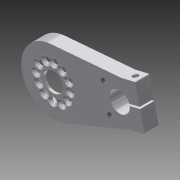
# Autodesk Inventor part: mount_alt
Saved by Autodesk Inventor 2015 SP1 (Build 190203100, 203)
## iProperties
Created: 2014-11-18
Part Number: mount_alt
Material: Aluminum 6061
Document SubType Name: Modeling
Designer: brent
Density: 2.7 g/cm^3
Appearance: Aluminum - Flat
Author: brent
Autodesk Inventor part; units mm, degrees
ref_plane "YZ Plane" through (0, 0, 0) normal (1, 0, 0) x (0, 1, 0)
ref_plane "XZ Plane" through (0, 0, 0) normal (0, 1, 0) x (-1, 0, 0)
ref_plane "XY Plane" through (0, 0, 0) normal (0, 0, 1) x (1, 0, 0)
derived "mount_sketch_alt.ipt"
sketch "Sketch2" plane through (0, 0, 0) normal (0, 0, 1) x (1, 0, 0)
  line L0 (72.4396, -72.2948) -> (-70.2441, 86.1715)
  line L1 (30.3736, -26.3701) -> (-42.626, -26.3701)
  circle A0 centre (-21.7992, 32.368) radius 3.9688
  circle A1 centre (-21.7992, 32.368) radius 9
  line L2 (-81.1368, 18.0799) -> (-21.7992, 32.368)
  circle A2 centre (-81.1368, 18.0799) radius 4
  circle A3 centre (-81.1368, 18.0799) radius 28.4798
  line L3 (-83.4978, 46.4616) -> (-7.6575, 52.7705)
  line L4 (-70.3199, -8.2657) -> (0.0796, 20.6388)
  line L5 (0.0796, 20.6388) -> (-7.6575, 52.7705)
  line L6 (-12.1479, 15.6185) -> (0.5521, 18.6766)
  line L7 (0.5521, 18.6766) -> (0.0796, 20.6388)
  line L8 (-12.8975, 33.695) -> (-3.6031, 35.933)
  line L9 (-13.2692, 35.2384) -> (-3.9747, 37.4764)
  line L10 (-88.9657, 5.285) -> (-93.9317, 25.9087)
  line L11 (-93.9317, 25.9087) -> (-73.308, 30.8748)
  line L12 (-73.308, 30.8748) -> (-68.3419, 10.251)
  line L13 (-68.3419, 10.251) -> (-88.9657, 5.285)
  line L14 (-88.9657, 5.285) -> (-73.308, 30.8748) construction
  line L15 (-93.9317, 25.9087) -> (-68.3419, 10.251) construction
  line L16 (-87.7302, 31.3952) -> (-67.3865, 25.3841)
  line L17 (-67.3865, 25.3841) -> (-73.3976, 5.0404)
  line L18 (-73.3976, 5.0404) -> (-93.7413, 11.0515)
  line L19 (-93.7413, 11.0515) -> (-87.7302, 31.3952)
  line L20 (-87.7302, 31.3952) -> (-73.3976, 5.0404) construction
  line L21 (-67.3865, 25.3841) -> (-93.7413, 11.0515) construction
  line L22 (-81.7046, 3.0401) -> (-96.3171, 18.4178)
  line L23 (-96.3171, 18.4178) -> (-80.9395, 33.0304)
  line L24 (-80.9395, 33.0304) -> (-66.3269, 17.6527)
  line L25 (-66.3269, 17.6527) -> (-81.7046, 3.0401)
  line L26 (-81.7046, 3.0401) -> (-80.9395, 33.0304) construction
  line L27 (-96.3171, 18.4178) -> (-66.3269, 17.6527) construction
  line L28 (-20.4639, 51.7052) -> (-8.1168, 54.6783)
  line L29 (-8.1168, 54.6783) -> (-7.6575, 52.7705)
  line L30 (-81.322, 18.0353) -> (-80.5639, 18.2178) construction
  line L31 (-79.3322, 9.7715) -> (-78.574, 9.954)
  line L32 (-82.5538, 26.4816) -> (-83.3119, 26.2991)
  arc A4 (-83.3119, 26.2991) -> (-79.3322, 9.7715) centre (-81.322, 18.0353) ccw
  arc A5 (-78.574, 9.954) -> (-82.5538, 26.4816) centre (-80.5639, 18.2178) ccw
  point P0 (0, 0)
  point P1 (-80.5639, 18.2178)
  point P2 (-80.943, 18.1265)
extrude "Extrusion1" add sketch "Sketch2" along normal blind 12.7 contours L6 L4 L0 | L0 L4 L7 L6 | L4 A3 L2 A1 L0 | L0 A1 L8 L5 L4 | A3 | L2 A3 L3 L0 A1 | L0 L3 L5 L9 A1 | L3 L28 L29 | L12 L24 L2 | L12 L17 L25 L13 L18 L22 L10 L19 L23 L11 L16 L24 | L2 L24 L17 L12 | L24 L12 L16 L17 L2 | L2 L17 L24 | L24 L16 L12 | L17 L24 L25 L12 | L12 L25 L17 | L16 L24 L11 L12 | L16 L11 L24 | L12 L13 L17 L25 | L17 L13 L25 | L16 L23 L24 L11 | L11 L23 L16 | L17 L18 L25 L13 | L25 L18 L13 | L23 L19 L11 | L11 L19 L16 L23 | L18 L25 L22 L13 | L13 L22 L18 | L19 L23 L10 L11 | L19 L10 L23 | L13 L10 L18 L22 | L18 L10 L22 | L19 L22 L23 L10 | L10 L22 L19 | L18 L19 L22 L10
sketch "Sketch3" plane through (-81.1368, 18.0799, 0) normal (0, 0, -1) x (-0.9722121, -0.2341019, 0)
  line L0 (-79.5587, -18.5434) -> (-79.5587, -0.7938) projected
  line L1 (-66.4957, -18.5434) -> (-79.5587, -18.5434) projected
  line L2 (-4.3488, -28.1458) -> (-66.4957, -18.5434) projected
  arc A0 (-4.3488, -28.1458) -> (-4.3488, 28.1458) centre (0, 0) ccw projected
  line L3 (-66.8587, 18.4873) -> (-4.3488, 28.1458) projected
  line L4 (-69.9986, 0.7937) -> (-79.5587, 0.7937) projected
  arc A1 (-69.9986, -0.7938) -> (-69.9986, 0.7937) centre (-61.0337, 0) ccw projected
  line L5 (-79.5587, -0.7938) -> (-69.9986, -0.7938) projected
  line L6 (0.6905, 0) -> (-0.6905, 0) construction
  line L7 (0.6905, 25.25) -> (-0.6905, 25.25)
  line L8 (-0.6905, -25.25) -> (0.6905, -25.25)
  arc A2 (0.6905, -25.25) -> (0.6905, 25.25) centre (0.6905, 0) ccw
  arc A3 (-0.6905, 25.25) -> (-0.6905, -25.25) centre (-0.6905, 0) ccw
  line L9 (-79.5587, 0.7937) -> (-79.5587, 18.4873) projected
  line L10 (-79.5587, 18.4873) -> (-66.8587, 18.4873) projected
  point P0 (-74.6497, -36.5717)
  dimension "d4" = 0.6905
  dimension "d5" = 50.5
  constraints: 8 end point, 4 point on circle, 4 tangent, 2 centre point, 1 horizontal, 1 midpoint, 1 parallel
  measures "d4" distance of A0.centre L6.end
  measures "d5" diameter of A3
extrude "Extrusion2" cut sketch "Sketch3" against normal blind 10.3188 contours A2 L8 A3 L7
hole "Hole1" at (-96.3171, 18.4178, 0) at (-93.7413, 11.0515, 0) at (-88.9657, 5.285, 0) at (-81.7046, 3.0401, 0) at (-73.3976, 5.0404, 0) at (-68.3419, 10.251, 0) at (-66.3269, 17.6527, 0) at (-67.3865, 25.3841, 0) at (-73.308, 30.8748, 0) at (-80.9395, 33.0304, 0) at (-87.7302, 31.3952, 0) at (-93.9317, 25.9087, 0) direction (0, 0, 1) diameter 4.3 end through all
sketch "Sketch4" plane through (0.5521, 18.6766, 0) normal (0.2341019, -0.9722121, 0) x (0.9722121, 0.2341019, 0)
  line L0 (-13.063, 0) -> (0, 0) projected
  line L1 (0, 0) -> (0, 12.7) projected
  line L2 (-13.063, 12.7) -> (0, 12.7) projected
  line L3 (-13.063, 0) -> (-13.063, 12.7) projected
  line L4 (-9.5601, 0) -> (-9.5601, 12.7) projected
  circle A0 centre (-6.0325, 6.35) radius 2.5527
  point P0 (-4.909, 0)
  dimension "d15" = 5.1054
  dimension "d17" = 6.0325
  dimension "d18" = 12.7
  dimension "d19" = 6.35
  constraints: 1 centre point
  measures "d15" diameter of A0
  measures "d17" distance from line of L1 A0.centre
  measures "d18" distance between parallel lines of L2 L0
  measures "d19" distance from line of L2 A0.centre
extrude "Extrusion3" cut sketch "Sketch4" against normal through all contours A0
ref_plane "Work Plane1" through (100.1901, 61.7421, 0) normal (0.2341019, -0.9722121, 0) x (0, 0, -1)
chamfer "Chamfer2" distance 2 angle 45 12 edges at (-87.7302, 29.2452, 12.7) (-80.9395, 30.8804, 12.7) (-73.308, 28.7248, 12.7) (-67.3865, 23.2341, 12.7) (-66.3269, 15.5027, 12.7) (-68.3419, 8.101, 12.7) (-73.3976, 2.8904, 12.7) (-81.7046, 0.8901, 12.7) (-88.9657, 3.135, 12.7) (-93.7413, 8.9015, 12.7) (-96.3171, 16.2678, 12.7) (-93.9317, 23.7587, 12.7)
sketch "Sketch8" plane through (-81.1368, 18.0799, 0) normal (0, 0, -1) x (-0.9722121, -0.2341019, 0)
  line L0 (-79.5587, -18.5434) -> (-79.5587, -0.7938) projected
  line L1 (-69.9986, 0.7937) -> (-79.5587, 0.7937) projected
  arc A0 (-69.9986, -0.7938) -> (-69.9986, 0.7937) centre (-61.0337, 0) ccw projected
  line L2 (-79.5587, -0.7938) -> (-69.9986, -0.7938) projected
  line L3 (-66.4957, -18.5434) -> (-79.5587, -18.5434) projected
  line L4 (-4.3488, -28.1458) -> (-66.4957, -18.5434) projected
  arc A1 (-4.3488, -28.1458) -> (-4.3488, 28.1458) centre (0, 0) ccw projected
  line L5 (-66.8587, 18.4873) -> (-4.3488, 28.1458) projected
  line L6 (-79.5587, 18.4873) -> (-66.8587, 18.4873) projected
  line L7 (-0.6905, 28.425) -> (0.6905, 28.425)
  arc A2 (0.6905, -28.425) -> (0.6905, 28.425) centre (0.6905, 0) ccw
  line L8 (0.6905, -28.425) -> (-0.6905, -28.425)
  arc A3 (-47.6803, -13.7402) -> (-47.6803, 13.7402) centre (-61.0337, 0) ccw
  line L9 (-47.6803, -13.7402) -> (-7.1186, -24.4181)
  line L10 (-47.6803, 13.7402) -> (-7.1186, 24.4181)
  arc A4 (-0.6905, 25.25) -> (-0.6905, -25.25) centre (-0.6905, 0) ccw projected
  line L11 (-79.5587, 0.7937) -> (-79.5587, 18.4873) projected
  point P0 (-74.6497, -36.5717)
  dimension "d55" = 10.16
  dimension "d91" = 7.62
  dimension "d92" = 7.62
  constraints: 8 end point, 6 point on circle, 2 centre point, 2 tangent
  measures "d55" radial gap between concentric circles of A0 A3
  measures "d91" distance from line of L5 L10.start
  measures "d92" distance from line of L4 L9.start
extrude "Extrusion6" cut sketch "Sketch8" against normal blind 6.35 contours A3 L10 A4 L9
fillet "Fillet6" radius 10.16 2 edges at (-37.9981, 42.6003, 3.175) (-31.5649, 15.8835, 3.175)
fillet "Fillet7" radius 12.7 2 edges at (-20.4639, 51.7052, 6.35) (-12.1479, 15.6185, 6.35)
sketch "Sketch13" plane through (-81.1368, 18.0799, 0) normal (0, 0, -1) x (-0.9722121, -0.2341019, 0)
  line L0 (-79.5587, -18.5434) -> (-79.5587, -0.7938) projected
  line L1 (-69.9986, 0.7937) -> (-79.5587, 0.7937) projected
  arc A0 (-69.9986, -0.7938) -> (-69.9986, 0.7937) centre (-61.0337, 0) ccw projected
  line L2 (-79.5587, -0.7938) -> (-69.9986, -0.7938) projected
  line L3 (-67.471, -18.5434) -> (-79.5587, -18.5434) projected
  arc A1 (-65.5317, -18.6924) -> (-67.471, -18.5434) centre (-67.471, -31.2434) ccw projected
  line L4 (-4.3488, -28.1458) -> (-65.5317, -18.6924) projected
  arc A2 (-4.3488, -28.1458) -> (-4.3488, 28.1458) centre (0, 0) ccw projected
  line L5 (-65.8947, 18.6363) -> (-4.3488, 28.1458) projected
  arc A3 (-67.834, 18.4873) -> (-65.8947, 18.6363) centre (-67.834, 31.1873) ccw projected
  line L6 (-79.5587, 18.4873) -> (-67.834, 18.4873) projected
  arc A4 (-0.6905, 25.25) -> (-0.6905, -25.25) centre (-0.6905, 0) ccw projected
  arc A5 (-0.6905, 25.25) -> (-7.1186, 24.4181) centre (-0.6905, 0) ccw projected
  line L7 (-0.6905, 25.25) -> (0.6905, 25.25) projected
  arc A6 (0.6905, -25.25) -> (0.6905, 25.25) centre (0.6905, 0) ccw projected
  line L8 (0.6905, -25.25) -> (-0.6905, -25.25) projected
  line L9 (-35.1982, 17.0261) -> (-7.1186, 24.4181) projected
  arc A7 (-7.1186, -24.4181) -> (-0.6905, -25.25) centre (-0.6905, 0) ccw projected
  line L10 (-7.1186, -24.4181) -> (-35.1982, -17.0261) projected
  arc A8 (-42.4605, -4.7056) -> (-35.1982, -17.0261) centre (-32.6117, -7.2008) ccw projected
  arc A9 (-42.4605, -4.7056) -> (-42.4605, 4.7056) centre (-61.0337, 0) ccw projected
  arc A10 (-35.1982, 17.0261) -> (-42.4605, 4.7056) centre (-32.6117, 7.2008) ccw projected
  line L11 (-79.5587, 0.7937) -> (-79.5587, 18.4873) projected
  point P0 (-74.6497, -36.5717)
extrude "Extrusion10" cut sketch "Sketch13" against normal blind 6.35 contours L7 A6 L8 A4 | A4 L10 A8 A9 A10 L9
fillet "Fillet10" radius 0.762 2 edges at (0.5521, 18.6766, 6.35) (-8.1168, 54.6783, 6.35)
sketch "Sketch17" plane through (-81.1368, 18.0799, 0) normal (0, 0, -1) x (-0.9722121, -0.2341019, 0)
  arc A0 (-69.9986, -0.7938) -> (-69.9986, 0.7937) centre (-61.0337, 0) ccw projected
  circle A1 centre (-61.0337, 0) radius 12.5
  arc A2 (-78.7967, 18.4873) -> (-79.5587, 17.7253) centre (-78.7967, 17.7253) ccw projected
  line L0 (-79.5587, 0.7937) -> (-79.5587, 17.7253) projected
  line L1 (-69.9986, 0.7937) -> (-79.5587, 0.7937) projected
  arc A3 (-69.9986, -0.7938) -> (-69.9986, 0.7937) centre (-61.0337, 0) ccw projected
  line L2 (-79.5587, -0.7938) -> (-69.9986, -0.7938) projected
  line L3 (-79.5587, -17.7814) -> (-79.5587, -0.7938) projected
  arc A4 (-79.5587, -17.7814) -> (-78.7967, -18.5434) centre (-78.7967, -17.7814) ccw projected
  line L4 (-67.471, -18.5434) -> (-78.7967, -18.5434) projected
  arc A5 (-65.5317, -18.6924) -> (-67.471, -18.5434) centre (-67.471, -31.2434) ccw projected
  line L5 (-4.3488, -28.1458) -> (-65.5317, -18.6924) projected
  arc A6 (-4.3488, -28.1458) -> (-4.3488, 28.1458) centre (0, 0) ccw projected
  line L6 (-65.8947, 18.6363) -> (-4.3488, 28.1458) projected
  arc A7 (-67.834, 18.4873) -> (-65.8947, 18.6363) centre (-67.834, 31.1873) ccw projected
  line L7 (-78.7967, 18.4873) -> (-67.834, 18.4873) projected
  circle A8 centre (-49.0787, 12.239) radius 2.413
  arc A9 (-0.6905, 25.25) -> (-7.1186, 24.4181) centre (-0.6905, 0) ccw projected
  line L8 (-0.6905, 25.25) -> (0.6905, 25.25) projected
  arc A10 (0.6905, -25.25) -> (0.6905, 25.25) centre (0.6905, 0) ccw projected
  line L9 (0.6905, -25.25) -> (-0.6905, -25.25) projected
  line L10 (-35.1982, 17.0261) -> (-7.1186, 24.4181) projected
  arc A11 (-7.1186, -24.4181) -> (-0.6905, -25.25) centre (-0.6905, 0) ccw projected
  line L11 (-7.1186, -24.4181) -> (-35.1982, -17.0261) projected
  arc A12 (-42.4605, -4.7056) -> (-35.1982, -17.0261) centre (-32.6117, -7.2008) ccw projected
  arc A13 (-42.4605, -4.7056) -> (-42.4605, 4.7056) centre (-61.0337, 0) ccw projected
  arc A14 (-35.1982, 17.0261) -> (-42.4605, 4.7056) centre (-32.6117, 7.2008) ccw projected
  point P0 (-74.6497, -36.5717)
  dimension "d93" = 25
  dimension "d94" = 4.826
  dimension "d95" = 8.89
  dimension "d101" = 30.48
  constraints: 2 centre point, 1 coincident
  measures "d93" diameter of A1
  measures "d94" diameter of A8
  measures "d95" distance from line of L6 A8.centre
  measures "d101" distance from line of L0 A8.centre
extrude "Extrusion11" cut sketch "Sketch17" against normal through all contours A8
thread "Thread2" size "10-32 UNF" class "2B" standard "ANSI Unified Screw Threads" full length
mirror "Mirror2" about plane through (100.1901, 61.7421, 0) normal (0.2341019, -0.9722121, 0) of "Extrusion11"
sketch "Sketch19" plane through (-81.1368, 18.0799, 0) normal (0, 0, -1) x (-0.9722121, -0.2341019, 0)
  circle A0 centre (-49.0787, -12.239) radius 2.413 projected
  circle A1 centre (-49.0787, 12.239) radius 2.413 projected
  arc A2 (-78.7967, 18.4873) -> (-79.5587, 17.7253) centre (-78.7967, 17.7253) ccw projected
  line L0 (-79.5587, 0.7937) -> (-79.5587, 17.7253) projected
  line L1 (-69.9986, 0.7937) -> (-79.5587, 0.7937) projected
  arc A3 (-69.9986, -0.7938) -> (-69.9986, 0.7937) centre (-61.0337, 0) ccw projected
  line L2 (-79.5587, -0.7938) -> (-69.9986, -0.7938) projected
  line L3 (-79.5587, -17.7814) -> (-79.5587, -0.7938) projected
  arc A4 (-79.5587, -17.7814) -> (-78.7967, -18.5434) centre (-78.7967, -17.7814) ccw projected
  line L4 (-67.471, -18.5434) -> (-78.7967, -18.5434) projected
  arc A5 (-65.5317, -18.6924) -> (-67.471, -18.5434) centre (-67.471, -31.2434) ccw projected
  line L5 (-4.3488, -28.1458) -> (-65.5317, -18.6924) projected
  arc A6 (-4.3488, -28.1458) -> (-4.3488, 28.1458) centre (0, 0) ccw projected
  line L6 (-65.8947, 18.6363) -> (-4.3488, 28.1458) projected
  arc A7 (-67.834, 18.4873) -> (-65.8947, 18.6363) centre (-67.834, 31.1873) ccw projected
  line L7 (-78.7967, 18.4873) -> (-67.834, 18.4873) projected
  line L8 (-35.1982, 17.0261) -> (-7.1186, 24.4181) projected
  arc A8 (-0.6905, 25.25) -> (-7.1186, 24.4181) centre (-0.6905, 0) ccw projected
  line L9 (-0.6905, 25.25) -> (0.6905, 25.25) projected
  arc A9 (0.6905, -25.25) -> (0.6905, 25.25) centre (0.6905, 0) ccw projected
  line L10 (0.6905, -25.25) -> (-0.6905, -25.25) projected
  arc A10 (-7.1186, -24.4181) -> (-0.6905, -25.25) centre (-0.6905, 0) ccw projected
  line L11 (-7.1186, -24.4181) -> (-35.1982, -17.0261) projected
  arc A11 (-42.4605, -4.7056) -> (-35.1982, -17.0261) centre (-32.6117, -7.2008) ccw projected
  arc A12 (-42.4605, -4.7056) -> (-42.4605, 4.7056) centre (-61.0337, 0) ccw projected
  arc A13 (-35.1982, 17.0261) -> (-42.4605, 4.7056) centre (-32.6117, 7.2008) ccw projected
  point P0 (-74.6497, -36.5717)
  dimension "d102" = 60.4444
  dimension "d103" = 61.2242
  dimension "d104" = 61.0337
  dimension "d105" = 108.7636
  constraints: 12 end point, 2 midpoint, 2 parallel, 2 point on line, 1 perpendicular, 1 point on circle, 4 other
equation "\"d19\" = 0.5 * d18"
body "Solid1"
